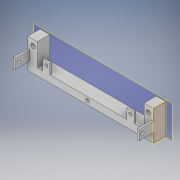
# Autodesk Inventor part: PC_bottom_piece
Saved by Autodesk Inventor 2017 (Build 210142000, 142)
## iProperties
Created: 2021-05-14
Part Number: PC_bottom_piece
Material: Generic
Document SubType Name: Modeling
Designer: Del
Density: 1 g/cm^3
Appearance: Default
Author: Del
Autodesk Inventor part; units mm, degrees
ref_plane "YZ Plane" through (0, 0, 0) normal (1, 0, 0) x (0, 1, 0)
ref_plane "XZ Plane" through (0, 0, 0) normal (0, 1, 0) x (-1, 0, 0)
ref_plane "XY Plane" through (0, 0, 0) normal (0, 0, 1) x (1, 0, 0)
sketch "Sketch1" plane through (0, 0, 0) normal (0, 0, 1) x (1, 0, 0)
  line L0 (0, 0) -> (0, 31.75)
  line L1 (0, 31.75) -> (10.16, 31.75)
  line L2 (10.16, 31.75) -> (10.16, 7.62)
  line L3 (10.16, 7.62) -> (15.748, 7.62)
  line L4 (15.748, 7.62) -> (15.748, 18.034)
  line L5 (15.748, 18.034) -> (23.368, 18.034)
  line L6 (23.368, 18.034) -> (23.368, 7.62)
  line L7 (23.368, 7.62) -> (105.283, 7.62)
  line L8 (105.283, 7.62) -> (105.283, 18.034)
  line L9 (105.283, 18.034) -> (112.903, 18.034)
  line L10 (112.903, 18.034) -> (112.903, 7.62)
  line L11 (112.903, 7.62) -> (123.571, 7.62)
  line L12 (123.571, 7.62) -> (123.571, 31.75)
  line L13 (123.571, 31.75) -> (133.731, 31.75)
  circle A0 centre (109.093, 14.224) radius 1.778
  circle A1 centre (5.588, 25.4) radius 1.905
  line L14 (133.731, 31.75) -> (133.731, 0)
  line L15 (133.731, 0) -> (0, 0)
  circle A2 centre (128.143, 25.4) radius 1.905
  circle A3 centre (19.558, 14.224) radius 1.778
  circle A4 centre (63.5, 4.064) radius 1.905
  dimension "d0" = 31.75
  dimension "d1" = 10.16
  dimension "d2" = 24.13
  dimension "d3" = 5.588
  dimension "d19" = 10.414
  dimension "d20" = 7.62
  dimension "d21" = 10.414
  dimension "d23" = 81.915
  dimension "d24" = 10.414
  dimension "d25" = 7.62
  dimension "d26" = 10.414
  dimension "d27" = 10.668
  dimension "d28" = 24.13
  dimension "d29" = 10.16
  dimension "d30" = 3.556
  dimension "d31" = 3.81
  dimension "d33" = 133.731
  dimension "d34" = 3.81
  dimension "d37" = 3.556
  dimension "d42" = 3.81
  dimension "d57" = 63.5
  dimension "d58" = 25.4
  constraints: 32 end point, 10 perpendicular, 5 centre point, 4 vertical, 1 horizontal
  measures "d0" distance of L0.start L0.end
  measures "d1" distance of L0.end L1.end
  measures "d2" distance of L1.end L2.end
  measures "d3" distance of L2.end L3.end
  measures "d19" distance of L3.end L4.end
  measures "d20" distance of L4.end L5.end
  measures "d21" distance of L5.end L6.end
  measures "d23" distance of L6.end L7.end
  measures "d24" distance of L7.end L8.end
  measures "d25" distance of L8.end L9.end
  measures "d26" distance of L9.end L10.end
  measures "d27" distance of L10.end L11.end
  measures "d28" distance of L11.end L12.end
  measures "d29" distance of L12.end L13.end
  measures "d30" diameter of A0
  measures "d31" diameter of A1
  measures "d33" distance of L14.end L0.start
  measures "d34" diameter of A2
  measures "d37" diameter of A3
  measures "d42" diameter of A4
  measures "d57" distance from line of A4.centre L0
  measures "d58" distance from line of A2.centre L15
sketch "Sketch2" plane through (0, 0, 0) normal (0, 0, 1) x (1, 0, 0)
  line L0 (15.748, 7.62) -> (10.16, 7.62) projected
  line L1 (12.954, 7.62) -> (117.9845, 7.62)
  line L2 (117.9845, 7.62) -> (117.9845, 21.0811)
  line L3 (117.9845, 21.0811) -> (12.954, 21.0811)
  line L4 (12.954, 21.0811) -> (12.954, 7.62)
  point P0 (0, 0)
  constraints: 8 end point, 2 parallel, 1 horizontal, 1 midpoint, 1 perpendicular
extrude "Extrusion4" add sketch "Sketch1" along normal blind 13.081
extrude "Extrusion5" cut sketch "Sketch2" along normal blind 11.176
sketch "Sketch3" plane through (0, 0, 0) normal (1, 0, 0) x (0, 1, 0)
  line L0 (31.75, 13.081) -> (0, 13.081) projected
  line L1 (19.9646, 13.081) -> (19.9646, 28.448)
  line L2 (19.9646, 28.448) -> (9.7883, 28.448)
  line L3 (9.7883, 28.448) -> (9.7883, 13.081)
  circle A0 centre (14.8765, 24.9237) radius 1.778
  point P0 (0, 0)
  dimension "d47" = 15.367
  dimension "d48" = 3.556
  constraints: 6 end point, 3 perpendicular, 2 point on line, 1 centre point
  measures "d47" distance of L1.start L1.end
  measures "d48" diameter of A0
extrude "Extrusion6" add sketch "Sketch3" along normal blind 2.032
ref_plane "Work Plane2" through (133.731, 0, 0) normal (1, 0, 0) x (0, 0, -1)
sketch "Sketch4" plane through (133.731, 0, 0) normal (1, 0, 0) x (0, 0, -1)
  line L0 (-13.081, 9.7883) -> (-28.448, 9.7883) projected
  line L1 (-28.448, 9.7883) -> (-28.448, 19.9646) projected
  line L2 (-13.081, 9.7883) -> (-28.448, 9.7883)
  line L3 (-28.448, 9.7883) -> (-28.448, 19.9646)
  line L4 (-28.448, 19.9646) -> (-13.081, 19.9646) projected
  line L5 (-28.448, 19.9646) -> (-13.081, 19.9646)
  line L6 (-13.081, 19.9646) -> (-13.081, 9.7883)
  line L7 (-13.081, 7.62) -> (-13.081, 18.034) projected
  circle A0 centre (-24.9237, 14.8765) radius 1.778 projected
  circle A1 centre (-24.9237, 14.8765) radius 1.778
  point P0 (0, 0)
  constraints: 8 end point, 2 collinear, 1 centre point, 1 coincident, 1 concentric, 1 horizontal, 1 perpendicular
extrude "Extrusion8" add sketch "Sketch4" against normal blind 2.032
ref_plane "Work Plane3" through (0, 0, 0) normal (0, 0, -1) x (-1, 0, 0)
sketch "Sketch5" plane through (0, 0, 0) normal (0, 0, -1) x (-1, 0, 0)
  circle A0 centre (-5.588, 25.4) radius 2.413
  circle A1 centre (-63.5, 4.064) radius 1.905 projected
  circle A2 centre (-63.5, 4.064) radius 2.286
  circle A3 centre (-128.1215, 25.4) radius 2.413
  point P0 (0, 0)
  dimension "d60" = 4.826
  dimension "d61" = 4.572
  dimension "d62" = 4.826
  constraints: 3 centre point, 1 coincident
  measures "d60" diameter of A0
  measures "d61" diameter of A2
  measures "d62" diameter of A3
extrude "Extrusion9" cut sketch "Sketch5" against normal blind 15.24 contours A0 | A1 | A3
body "Solid2"
body "Solid3"
